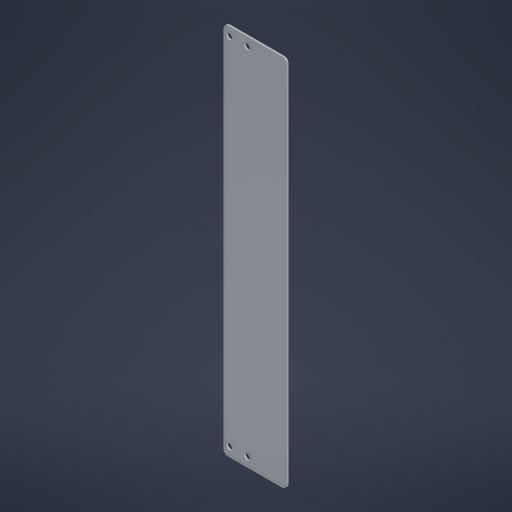
# Autodesk Inventor part: wingplexi
Saved by Autodesk Inventor 2023 (Build 270158000, 158)
## iProperties
Created: 2023-08-07
Part Number: wingplexi
Material: Generic
Document SubType Name: Modeling
Designer: srbel
Density: 1 g/cm^3
Appearance: Clear - White
Author: srbel
Autodesk Inventor part; units mm, degrees
ref_plane "YZ Plane" through (0, 0, 0) normal (1, 0, 0) x (0, 1, 0)
ref_plane "XZ Plane" through (0, 0, 0) normal (0, 1, 0) x (-1, 0, 0)
ref_plane "XY Plane" through (0, 0, 0) normal (0, 0, 1) x (1, 0, 0)
sketch "Sketch1" plane through (0, 0, 0) normal (0, 0, 1) x (1, 0, 0)
  circle A0 centre (3.9687, -260.35) radius 2.1844
  circle A1 centre (16.6687, -260.35) radius 2.1844
  circle A2 centre (3.9687, -6.35) radius 2.1844
  circle A3 centre (16.6687, -6.35) radius 2.1844
  line L0 (3.175, -266.7) -> (8.0073, -266.7)
  line L1 (12.6301, -266.7) -> (20.6375, -266.7)
  line L2 (41.8702, 0) -> (3.175, 0)
  line L3 (3.175, -266.7) -> (41.8702, -266.7)
  line L4 (45.0452, -263.525) -> (45.0452, -3.175)
  line L5 (41.8702, 0) -> (3.175, 0)
  line L6 (0, -3.175) -> (0, -263.525)
  circle A4 centre (3.9687, -260.35) radius 2.1844
  circle A5 centre (16.6687, -260.35) radius 2.1844
  circle A6 centre (3.9687, -6.35) radius 2.1844
  circle A7 centre (16.6687, -6.35) radius 2.1844
  arc A8 (41.8702, -266.7) -> (45.0452, -263.525) centre (41.8702, -263.525) ccw
  arc A9 (0, -263.525) -> (3.175, -266.7) centre (3.175, -263.525) ccw
  arc A10 (3.175, 0) -> (0, -3.175) centre (3.175, -3.175) ccw
  arc A11 (45.0452, -3.175) -> (41.8702, 0) centre (41.8702, -3.175) ccw
  point P0 (0, 0)
  dimension "d0" = 3.175
  constraints: 14 end point, 12 centre point, 8 point on circle, 8 tangent, 7 equal radius, 4 coincident, 1 perpendicular
  measures "d0" radius of A8
extrude "Extrusion1" add sketch "Sketch1" along normal blind 1.5875
body "Solid1"
